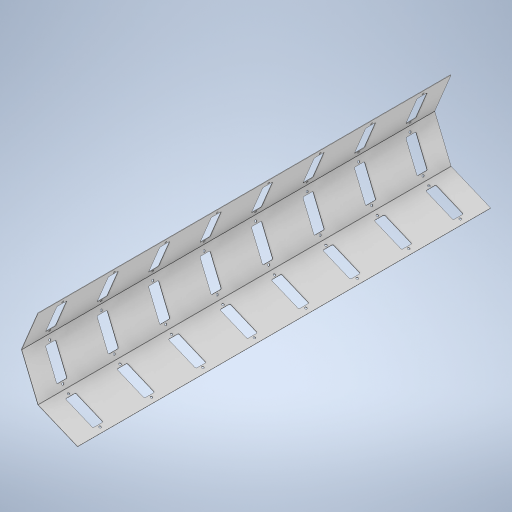
# Autodesk Inventor part: ДМФ 01 13 Барабан Лист лев брт
Saved by Autodesk Inventor 2024.2 (Build 282272000, 272)
## iProperties
Created: 2024-04-28
Part Number: ДМФ 01 13 Барабан Лист лев брт
Material: Generic
Document SubType Name: Sheet Metal
Designer: pokla
Density: 1 g/cm^3
Appearance: Default
Sheet Metal Rule: Default
Flat Pattern Width: 62.4873 cm
Flat Pattern Length: 200.6 cm
Flat Pattern Area: 12534.9 cm^2
Sheet Metal Width: 624,873 mm
Sheet Metal Length: 2006,000 mm
Sheet Metal Area: 1253494,564 mm^2
Author: pokla
Autodesk Inventor part; units mm, degrees
ref_plane "YZ Plane" through (0, 0, 0) normal (1, 0, 0) x (0, 1, 0)
ref_plane "XZ Plane" through (0, 0, 0) normal (0, 1, 0) x (-1, 0, 0)
ref_plane "XY Plane" through (0, 0, 0) normal (0, 0, 1) x (1, 0, 0)
sketch "Sketch2" plane through (0, 0, 0) normal (0, 0, 1) x (1, 0, 0)
  line L0 (0, 273.8452) -> (193.6378, 193.6378) construction
  line L1 (193.6378, 193.6378) -> (273.8452, 0) construction
  line L2 (273.8452, 0) -> (193.6378, -193.6378) construction
  line L3 (193.6378, -193.6378) -> (0, -273.8452) construction
  line L4 (0, -273.8452) -> (-193.6378, -193.6378) construction
  line L5 (-193.6378, -193.6378) -> (-273.8452, 0) construction
  line L6 (-273.8452, 0) -> (-193.6378, 193.6378) construction
  line L7 (-193.6378, 193.6378) -> (0, 273.8452) construction
  line L8 (-273.2112, -1.5307) -> (-194.2719, -192.1071)
  line L9 (-192.1071, -194.2719) -> (-0.8315, -273.5008)
  arc A0 (-273.2112, 1.5307) -> (-273.2112, -1.5307) centre (-269.5157, 0) ccw
  arc A1 (-194.2719, -192.1071) -> (-192.1071, -194.2719) centre (-190.5763, -190.5763) ccw
  line L10 (-273.2112, 1.5307) -> (-193.9822, 192.8063)
  point P0 (0, 0)
  point P1 (0, 0)
  dimension "d58" = 4
  dimension "d59" = 4
  dimension "d70" = 0.9
  dimension "d72" = 0.9
  dimension "d74" = 506
  measures "d58" radius of A0
  measures "d59" radius of A1
  measures "d70" distance of L3.end L9.end
  measures "d72" distance of L6.end L10.end
  measures "d74" distance between parallel lines of L1 L8
contour flange "Contour Flange3" sketch "Sketch2" thickness 2 bend radius 2 width 2006 along (0, 0, -1) mid plane no both sides no wall seen from (-96.4693, -233.8863, 0) lies toward (0.3826834, 0.9238795, 0) curves L9 A1 L8 A0 L10
bend "Bend6"
corner "Corner6"
sketch "Sketch11" plane through (-271.3634, -0.7654, 0) normal (0.9238795, 0.3826834, 0) x (0, 0, -1)
  line L0 (0, 0) -> (2006, 0) projected
  line L1 (0, -206.2784) -> (0, 0) projected
  line L2 (0, -206.2784) -> (2006, -206.2784) projected
  line L3 (2006, -206.2784) -> (2006, 0) projected
  circle A0 centre (878, -20.6392) radius 5
  circle A1 centre (878, -185.6392) radius 5
  line L4 (853, -30.6392) -> (903, -30.6392)
  line L5 (903, -30.6392) -> (903, -175.6392)
  line L6 (903, -175.6392) -> (853, -175.6392)
  line L7 (853, -175.6392) -> (853, -30.6392)
  line L8 (853, -103.1392) -> (903, -103.1392) construction
  point P0 (0, -103.1392)
  point P1 (2006, -103.1392)
  point P2 (878, -30.6392)
  point P3 (878, -175.6392)
  point P4 (1003, 0)
  dimension "d141" = 50
  dimension "d142" = 145
  dimension "d143" = 10
  dimension "d145" = 125
  dimension "d146" = 10
  constraints: 10 end point, 6 midpoint, 2 centre point, 2 horizontal, 2 parallel, 2 vertical alignment, 1 equal radius, 1 horizontal alignment, 1 perpendicular, 1 other
  measures "d141" distance of L4.start L4.end
  measures "d142" distance of L4.end L5.end
  measures "d143" distance from line of A0.centre L4
  measures "d145" horizontal distance of A0.centre point (1003, 0)
  measures "d146" diameter of A0
extrude "Extrusion4" cut sketch "Sketch11" against normal blind 10 contours A0 | A1 | L4 L5 L6 L7
fillet "Fillet1" radius 5 4 edges at (-260.5622, -29.455, -903) (-260.5622, -29.455, -853) (-205.0731, -163.4175, -853) (-205.0731, -163.4175, -903)
pattern_circular "Circular Pattern2" count 3 over 90 about axis through (0, 0, -10) along (0, 0, 1) of "Extrusion4", "Fillet1" both ways yes
pattern_linear "Rectangular Pattern2" count 8 spacing 250 along (0, 0, -1) of "Extrusion4", "Fillet1", "Circular Pattern2" first direction both ways yes
fillet "Corner Round1" radius 2 1 edges at (-193.0584, 192.4236, -2006)
equation "\"d58\" = BendRadius + Thickness"
equation "\"d59\" = BendRadius + Thickness"
equation "\"d74\" = Барабан_габарит_по_кассетам"
equation "\"d75\" = Thickness"
equation "\"d76\" = BendReliefWidth"
equation "\"d77\" = BendReliefDepth"
equation "\"d78\" = MinimumRemnant"
equation "\"d79\" = TransitionRadius"
equation "\"d80\" = Барабан_длина_листа"
equation "\"d81\" = BendRadius"
equation "\"d83\" = CornerReliefSize"
equation "\"d84\" = GapSize"
equation "\"d85\" = JacobiRadiusSize"
equation "\"BendRadius\" = Thickness"
equation "\"BendReliefWidth\" = Thickness"
equation "\"BendReliefDepth\" = 0.5 * Thickness"
equation "\"CornerReliefSize\" = 4 * Thickness"
equation "\"MinimumRemnant\" = 2 * Thickness"
equation "\"TransitionRadius\" = BendRadius"
equation "\"JacobiRadiusSize\" = BendRadius"
equation "\"GapSize\" = Thickness"
equation "\"Thickness\" = 2"
equation "\"Барабан_габарит_по_кассетам\" = 506"
equation "\"Барабан_длина_листа\" = 2006"
body "Solid3"
